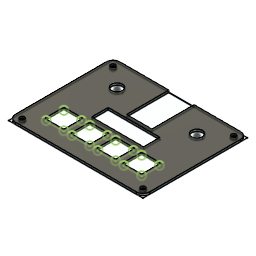
Assembly Hackerpad (Autodesk Fusion 360 archive; units mm, degrees)
design "top plate"
Autodesk Fusion 360 part; units mm, degrees
sketch "plate-2026-01-04T06_23_53.757Z" plane through (0, 0, 0) normal (0, 0, 1) x (1, 0, 0)
  line L0 (3.025, -40.625) -> (16.025, -40.625)
  line L1 (3.025, -54.625) -> (16.025, -54.625)
  line L2 (2.525, -41.125) -> (2.525, -54.125)
  line L3 (16.525, -41.125) -> (16.525, -54.125)
  arc A0 (3.025, -40.625) -> (2.525, -41.125) centre (3.025, -41.125) ccw
  arc A1 (16.525, -41.125) -> (16.025, -40.625) centre (16.025, -41.125) ccw
  arc A2 (2.525, -54.125) -> (3.025, -54.625) centre (3.025, -54.125) ccw
  arc A3 (16.025, -54.625) -> (16.525, -54.125) centre (16.025, -54.125) ccw
  line L4 (22.075, -40.625) -> (35.075, -40.625)
  line L5 (22.075, -54.625) -> (35.075, -54.625)
  line L6 (21.575, -41.125) -> (21.575, -54.125)
  line L7 (35.575, -41.125) -> (35.575, -54.125)
  arc A4 (22.075, -40.625) -> (21.575, -41.125) centre (22.075, -41.125) ccw
  arc A5 (35.575, -41.125) -> (35.075, -40.625) centre (35.075, -41.125) ccw
  arc A6 (21.575, -54.125) -> (22.075, -54.625) centre (22.075, -54.125) ccw
  arc A7 (35.075, -54.625) -> (35.575, -54.125) centre (35.075, -54.125) ccw
  line L8 (41.125, -40.625) -> (54.125, -40.625)
  line L9 (41.125, -54.625) -> (54.125, -54.625)
  line L10 (40.625, -41.125) -> (40.625, -54.125)
  line L11 (54.625, -41.125) -> (54.625, -54.125)
  arc A8 (41.125, -40.625) -> (40.625, -41.125) centre (41.125, -41.125) ccw
  arc A9 (54.625, -41.125) -> (54.125, -40.625) centre (54.125, -41.125) ccw
  arc A10 (40.625, -54.125) -> (41.125, -54.625) centre (41.125, -54.125) ccw
  arc A11 (54.125, -54.625) -> (54.625, -54.125) centre (54.125, -54.125) ccw
  line L12 (60.175, -40.625) -> (73.175, -40.625)
  line L13 (60.175, -54.625) -> (73.175, -54.625)
  line L14 (59.675, -41.125) -> (59.675, -54.125)
  line L15 (73.675, -41.125) -> (73.675, -54.125)
  arc A12 (60.175, -40.625) -> (59.675, -41.125) centre (60.175, -41.125) ccw
  arc A13 (73.675, -41.125) -> (73.175, -40.625) centre (73.175, -41.125) ccw
  arc A14 (59.675, -54.125) -> (60.175, -54.625) centre (60.175, -54.125) ccw
  arc A15 (73.175, -54.625) -> (73.675, -54.125) centre (73.175, -54.125) ccw
  line L16 (-10.823, 8.872) -> (87.977, 8.872)
  line L17 (87.977, 8.872) -> (87.977, -67.928)
  line L18 (87.977, -67.928) -> (-10.823, -67.928)
  line L19 (-10.823, -67.928) -> (-10.823, 8.872)
  circle A16 centre (-5.823, 3.872) radius 1.7
  circle A17 centre (82.977, 3.872) radius 1.7
  circle A18 centre (82.977, -62.928) radius 1.7
  circle A19 centre (-5.823, -62.928) radius 1.7
  line L20 (30.232, 8.872) -> (48.732, 8.872)
  line L21 (48.732, 8.872) -> (48.732, -22.128)
  line L22 (48.732, -22.128) -> (30.232, -22.128)
  line L23 (30.232, -22.128) -> (30.232, 8.872)
  circle A20 centre (9.427, -8.428) radius 4
  circle A21 centre (68.227, -8.428) radius 4
  line L24 (18.992, -24.543) -> (56.992, -24.543)
  line L25 (56.992, -24.543) -> (56.992, -36.543)
  line L26 (56.992, -36.543) -> (18.992, -36.543)
  line L27 (18.992, -36.543) -> (18.992, -24.543)
  dimension "d1" = 76.8
  dimension "d2" = 98.8
  dimension "d3" = 13.348
  dimension "d4" = 13.303
  dimension "d5" = 3.4
  dimension "d6" = 5
  dimension "d7" = 5
  dimension "d8" = 3.4
  dimension "d9" = 5
  dimension "d10" = 5
  dimension "d11" = 3.4
  dimension "d12" = 5
  dimension "d13" = 5
  dimension "d14" = 3.4
  dimension "d15" = 5
  dimension "d16" = 5
  dimension "d17" = 31
  dimension "d18" = 18.5
  dimension "d19" = 41.055
  dimension "d20" = 8
  dimension "d21" = 17.3
  dimension "d22" = 20.25
  dimension "d23" = 8
  dimension "d24" = 17.3
  dimension "d25" = 19.75
  dimension "d26" = 12
  dimension "d27" = 38
  dimension "d28" = 29.815
  dimension "d29" = 31.385
  constraint horizontal L16
  constraint vertical L17
  constraint horizontal L18
  constraint vertical L19
  constraint horizontal L20
  constraint vertical L21
  constraint horizontal L22
  constraint vertical L23
  constraint coincident L16 L20.start
  constraint horizontal L24
  constraint vertical L25
  constraint horizontal L26
  constraint vertical L27
  measures "d1" distance of L16.start L18.end
  measures "d2" distance of L16.start L16.end
  measures "d3" distance of L2 L19
  measures "d4" distance of L1 L18
  measures "d5" diameter of A16
  measures "d6" distance of L16 A16.centre
  measures "d7" distance of L19 A16.centre
  measures "d8" diameter of A17
  measures "d9" distance of L16 A17.centre
  measures "d10" distance of L17 A17.centre
  measures "d11" diameter of A18
  measures "d12" distance of L17 A18.centre
  measures "d13" distance of L18 A18.centre
  measures "d14" diameter of A19
  measures "d15" distance of L19 A19.centre
  measures "d16" distance of L18 A19.centre
  measures "d17" distance of L20.start L22.end
  measures "d18" distance of L21.end L22.end
  measures "d19" distance of L19 L23
  measures "d20" diameter of A20
  measures "d21" distance of L16 A20.centre
  measures "d22" distance of L19 A20.centre
  measures "d23" diameter of A21
  measures "d24" distance of L16 A21.centre
  measures "d25" distance of L17 A21.centre
  measures "d26" distance of L24.start L26.end
  measures "d27" distance of L24.start L24.end
  measures "d28" distance of L19 L27
  measures "d29" distance of L18 L26
extrude "Extrude1" add sketch "plate-2026-01-04T06_23_53.757Z" along normal blind 1.5 contours L16 L17 L18 L19 L21 L22 L23
fillet "Fillet1" radius 5 1 edges at (87.977, 8.872, 0.75)
fillet "Fillet2" radius 5 1 edges at (-10.823, 8.872, 0.75)
fillet "Fillet3" radius 5 1 edges at (-10.823, -67.928, 0.75)
fillet "Fillet4" radius 5 1 edges at (87.977, -67.928, 0.75)
equation "d3 = 9.5 mm + 3.848 mm"
equation "d4 = 3.803 mm + 9.5 mm"
equation "d19 = 35.305 mm + 5.75 mm"
equation "d21 = 7.8 mm + 9.5 mm"
equation "d22 = 9.5 mm + 10.75 mm"
equation "d24 = 9.5 mm + 7.8 mm"
equation "d25 = 9.5 mm + 10.250 mm"
equation "d28 = 9.5 mm + 20.315 mm"
equation "d29 = 21.885 mm + 9.5 mm"
